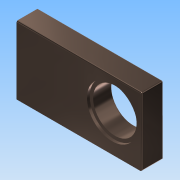
# Autodesk Inventor part: держатель шкивов 2
Saved by Autodesk Inventor 2017 (Build 210142000, 142)
## iProperties
Part Number: держатель шкивов 2
Material: Типовые
Document SubType Name: Modeling
Designer: Max
Mass: 7.38695 g
Surface Area: 35.2469 cm^2
Volume: 7.38695 cm^3
Density: 1 g/cm^3
Appearance: Оружейный металл — антик — полированный
Author: Max
Autodesk Inventor part; units mm, degrees
ref_plane "YZ Plane" through (0, 0, 0) normal (1, 0, 0) x (0, 1, 0)
ref_plane "XZ Plane" through (0, 0, 0) normal (0, 1, 0) x (-1, 0, 0)
ref_plane "XY Plane" through (0, 0, 0) normal (0, 0, 1) x (1, 0, 0)
sketch "Эскиз1" plane through (0, 0, 0) normal (0, 1, 0) x (-1, 0, 0)
  line L0 (0, 0) -> (46, 0)
  line L1 (46, 0) -> (46, -25)
  line L2 (46, -25) -> (0, -25)
  line L3 (0, -25) -> (0, 0)
  circle A0 centre (10.8656, -11.5046) radius 8
  circle A1 centre (10.8656, -11.5046) radius 9.25
  dimension "d0" = 25
  dimension "d1" = 46
  dimension "d2" = 16
  dimension "d3" = 18.5
  constraints: 8 end point, 2 centre point, 2 parallel, 1 coincident, 1 horizontal, 1 perpendicular
  measures "d0" distance between parallel lines of L2 L0
  measures "d1" distance between parallel lines of L3 L1
  measures "d2" diameter of A0
  measures "d3" diameter of A1
extrude "Выдавливание1" add sketch "Эскиз1" along normal blind 8 contours L0 L1 L2 L3 | A1
extrude "Выдавливание2" cut sketch "Эскиз1" along normal blind 1 contours A1
sketch "Эскиз2" plane through (-46, 0, -25) normal (-1, 0, 0) x (0, 0, 1)
  line L0 (0, 0) -> (0, 8) projected
  line L1 (0, 4) -> (25, 4) construction
  line L2 (25, 0) -> (25, 8) projected
  circle A0 centre (13.1, 4) radius 2
  dimension "d8" = 4
  dimension "d15" = 13.1
  constraints: 2 end point, 2 midpoint, 1 centre point, 1 point on line
  measures "d8" diameter of A0
  measures "d15" distance from line of L0 A0.centre
sketch "Эскиз3" plane through (0, 0, -25) normal (0, 0, -1) x (-1, 0, 0)
  line L0 (46, 0) -> (46, 8) projected
  line L1 (46, 4) -> (17.4, 4)
  circle A0 centre (17.4, 4) radius 2
  point P0 (0, 0)
  dimension "d9" = 4
  dimension "d14" = 28.6
  constraints: 2 end point, 1 centre point, 1 coincident, 1 horizontal, 1 midpoint
  measures "d9" diameter of A0
  measures "d14" distance from line of L0 L1.end
extrude "Выдавливание3" cut sketch "Эскиз3" against normal blind 5
extrude "Выдавливание4" cut sketch "Эскиз2" against normal blind 5
fillet "Сопряжение1" radius 0.5 6 edges at (0, 0, -12.5) (0, 8, -12.5) (0, 4, 0) (0, 4, -25) (-23, 8, 0) (-23, 0, 0)
fillet "Сопряжение2" radius 0.5 1 edges at (-2.8656, 8, -11.5046)
